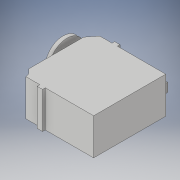
# Autodesk Inventor part: DS3218_motor
Saved by Autodesk Inventor 2018 (Build 220112000, 112)
## iProperties
Created: 2020-03-26
Part Number: DS3218_motor
Material: Generic
Document SubType Name: Modeling
Designer: natha
Density: 1 g/cm^3
Appearance: Default
Author: natha
Autodesk Inventor part; units mm, degrees
ref_plane "YZ Plane" through (0, 0, 0) normal (1, 0, 0) x (0, 1, 0)
ref_plane "XZ Plane" through (0, 0, 0) normal (0, 1, 0) x (-1, 0, 0)
ref_plane "XY Plane" through (0, 0, 0) normal (0, 0, 1) x (1, 0, 0)
sketch "Sketch1" plane through (0, 0, 0) normal (0, 1, 0) x (-1, 0, 0)
  line L0 (0, 0) -> (40.8, 0)
  line L1 (40.8, 0) -> (40.8, -40.25)
  line L2 (40.8, -40.25) -> (0, -40.25)
  line L3 (0, -40.25) -> (0, 0)
  dimension "d0" = 40.8
  dimension "d1" = 40.25
  constraints: 8 end point, 2 parallel, 1 horizontal, 1 perpendicular
  measures "d0" distance of L1.end L2.end
  measures "d1" distance of L0.end L1.end
extrude "Extrusion1" add sketch "Sketch1" along normal blind 20.35
sketch "Sketch2" plane through (0, 20.35, 0) normal (0, 1, 0) x (1, 0, 0)
  line L0 (-40.8, 0) -> (0, 0) projected
  line L1 (-40.8, 0) -> (-40.8, 4.68)
  line L2 (-40.8, 40.25) -> (-40.8, 0) projected
  line L3 (-40.8, 0) -> (-37.8, 0)
  line L4 (-37.8, 0) -> (-38.396, 2.1177)
  line L5 (-38.396, 2.1177) -> (-40.8, 4.68)
  dimension "d4" = 4.68
  dimension "d5" = 3
  dimension "d6" = 2.2
  constraints: 8 end point, 2 point on line
  measures "d4" distance of L0.start L1.end
  measures "d5" distance of L0.start L3.end
  measures "d6" distance of L3.end L4.end
extrude "Extrusion2" cut sketch "Sketch2" against normal blind 20.35
sketch "Sketch3" plane through (0, 20.35, 0) normal (0, 1, 0) x (1, 0, 0)
  line L0 (-40.8, 4.68) -> (-40.8, 40.25) projected
  line L1 (-40.8, 40.25) -> (-36.8, 40.25)
  line L2 (-40.8, 40.25) -> (0, 40.25) projected
  line L3 (-40.8, 40.25) -> (-40.8, 35.25)
  line L4 (-40.8, 35.25) -> (-36.8, 40.25)
  point P0 (0, 0)
  dimension "d9" = 4
  dimension "d10" = 5
  constraints: 6 end point, 1 horizontal, 1 point on line
  measures "d9" distance of L0.end L1.end
  measures "d10" distance of L0.end L3.end
extrude "Extrusion3" cut sketch "Sketch3" against normal blind 20.35
sketch "Sketch4" plane through (-40.8, 0, -4.68) normal (-1, 0, 0) x (0, 0, 1)
  circle A0 centre (-25.57, 10.175) radius 2.625
  line L0 (-35.57, 0) -> (-35.57, 20.35) projected
  line L1 (-30.57, 20.35) -> (0, 20.35) projected
  point P0 (4.68, 0)
  dimension "d13" = 5.25
  dimension "d14" = 10
  dimension "d15" = 10.175
  constraints: 1 centre point
  measures "d13" diameter of A0
  measures "d14" distance from line of L0 A0.centre
  measures "d15" distance from line of L1 A0.centre
extrude "Extrusion4" add sketch "Sketch4" along normal blind 1.5
sketch "Sketch5" plane through (-42.3, 10.175, -30.25) normal (-1, 0, 0) x (0, 0, 1)
  circle A0 centre (0, 0) radius 4.375
  point P0 (30.25, -10.175)
  dimension "d18" = 8.75
  constraints: 1 centre point
  measures "d18" diameter of A0
extrude "Extrusion5" add sketch "Sketch5" along normal blind 2.8
sketch "Sketch6" plane through (-45.1, 10.175, -30.25) normal (-1, 0, 0) x (0, 0, 1)
  circle A0 centre (0, 0) radius 10
  point P0 (30.25, -10.175)
  dimension "d21" = 20
  constraints: 1 centre point
  measures "d21" diameter of A0
extrude "Extrusion6" add sketch "Sketch6" along normal blind 2.2
sketch "Sketch7" plane through (0, 0, 0) normal (0, 0, 1) x (1, 0, 0)
  line L0 (-7, 6.875) -> (-3.25, 6.875)
  line L1 (-3.25, 6.875) -> (-3.25, 13.475)
  line L2 (-3.25, 13.475) -> (-7, 13.475)
  line L3 (-7, 13.475) -> (-7, 6.875)
  line L4 (0, 0) -> (0, 20.35) projected
  line L5 (0, 0) -> (-37.8, 0) projected
  dimension "d24" = 3.75
  dimension "d25" = 6.6
  dimension "d26" = 7
  dimension "d27" = 6.875
  constraints: 8 end point, 2 parallel, 1 horizontal, 1 perpendicular
  measures "d24" distance of L2.end L1.end
  measures "d25" distance of L1.end L0.end
  measures "d26" distance between parallel lines of L3 L4
  measures "d27" distance between parallel lines of L5 L0
extrude "Extrusion7" add sketch "Sketch7" along normal blind 4.5
chamfer "Chamfer1" distance 2 angle 45 2 edges at (-5.125, 13.475, 4.5) (-5.125, 6.875, 4.5)
sketch "Sketch8" plane through (-7, 6.875, 0) normal (-1, 0, 0) x (0, 0, 1)
  line L0 (0, 6.6) -> (0, 0) projected
  line L1 (0, 0) -> (0, 6.6)
  line L2 (0, 6.6) -> (2.5, 6.6) projected
  line L3 (0, 6.6) -> (2.5, 6.6)
  line L4 (4.5, 4.6) -> (4.5, 2) projected
  line L5 (2.5, 6.6) -> (4.5, 4.6)
  line L6 (4.5, 4.6) -> (4.5, 2)
  line L7 (4.5, 2) -> (2.5, 0) projected
  line L8 (4.5, 2) -> (2.5, 0)
  line L9 (0, 0) -> (2.5, 0) projected
  line L10 (2.5, 0) -> (0, 0)
  point P0 (0, -6.875)
  constraints: 12 end point, 2 parallel, 1 collinear, 1 perpendicular, 1 vertical
extrude "Extrusion8" cut sketch "Sketch8" against normal blind 4.5
sketch "Sketch9" plane through (0, 0, -40.25) normal (0, 0, -1) x (-1, 0, 0)
  line L0 (3.25, 6.875) -> (7, 6.875)
  line L1 (7, 6.875) -> (7, 13.475)
  line L2 (7, 13.475) -> (3.25, 13.475)
  line L3 (3.25, 13.475) -> (3.25, 6.875)
  line L4 (0, 20.35) -> (36.8, 20.35) projected
  line L5 (0, 0) -> (0, 20.35) projected
  dimension "d35" = 3.75
  dimension "d36" = 6.6
  dimension "d37" = 6.875
  dimension "d45" = 7
  constraints: 8 end point, 2 parallel, 1 horizontal, 1 perpendicular
  measures "d35" distance of L2.end L1.end
  measures "d36" distance of L1.end L0.end
  measures "d37" distance between parallel lines of L4 L2
  measures "d45" distance between parallel lines of L1 L5
extrude "Extrusion9" add sketch "Sketch9" along normal blind 4.5
chamfer "Chamfer2" distance 1 angle 45 2 edges at (-5.125, 6.875, -44.75) (-5.125, 13.475, -44.75)
sketch "Sketch10" plane through (-7, 6.875, -40.25) normal (-1, 0, 0) x (0, 0, 1)
  line L0 (0, 0) -> (0, 6.6) projected
  line L1 (-4.5, 1) -> (-4.5, 5.6) projected
  line L2 (0, 0) -> (-4.5, 1)
  line L3 (0, 0) -> (-3.5, 0) projected
  line L4 (-4.5, 1) -> (-3.5, 0)
  line L5 (-3.5, 0) -> (0, 0)
  line L6 (0, 6.6) -> (-3.5, 6.6) projected
  line L7 (-4.5, 5.6) -> (-3.5, 6.6)
  line L8 (-3.5, 6.6) -> (0, 6.6)
  line L9 (0, 6.6) -> (-4.5, 5.6)
  point P0 (40.25, -6.875)
  constraints: 12 end point, 2 collinear
extrude "Extrusion10" cut sketch "Sketch10" against normal blind 4.5 contours L3 L4 L2 | L9 L7 L6
sketch "Sketch11" plane through (0, 0, -40.25) normal (0, 0, -1) x (-1, 0, 0)
  line L0 (0, 20.35) -> (36.8, 20.35) projected
  line L1 (27, 0) -> (30, 0)
  line L2 (30, 0) -> (30, 20.35)
  line L3 (30, 20.35) -> (27, 20.35)
  line L4 (27, 20.35) -> (27, 0)
  line L5 (0, 0) -> (0, 20.35) projected
  dimension "d46" = 3
  dimension "d47" = 27
  constraints: 8 end point, 2 parallel, 1 horizontal, 1 perpendicular, 1 point on line
  measures "d46" distance of L3.end L2.end
  measures "d47" distance between parallel lines of L5 L4
extrude "Extrusion11" add sketch "Sketch11" along normal blind 1.5
sketch "Sketch12" plane through (0, 0, 0) normal (0, 0, 1) x (1, 0, 0)
  line L0 (0, 0) -> (-37.8, 0) projected
  line L1 (0, 20.35) -> (-27, 20.35) projected
  line L2 (-27, 0) -> (-30, 0)
  line L3 (-30, 0) -> (-30, 20.35)
  line L4 (-30, 20.35) -> (-27, 20.35)
  line L5 (-27, 20.35) -> (-27, 0)
  line L6 (0, 0) -> (0, 20.35) projected
  dimension "d50" = 3
  dimension "d51" = 27
  constraints: 8 end point, 2 parallel, 2 point on line, 1 horizontal, 1 perpendicular
  measures "d50" distance of L3.end L4.end
  measures "d51" distance between parallel lines of L6 L5
extrude "Extrusion12" add sketch "Sketch12" along normal blind 1.5 contours L0 L3 L4 L5
body "Solid1"
